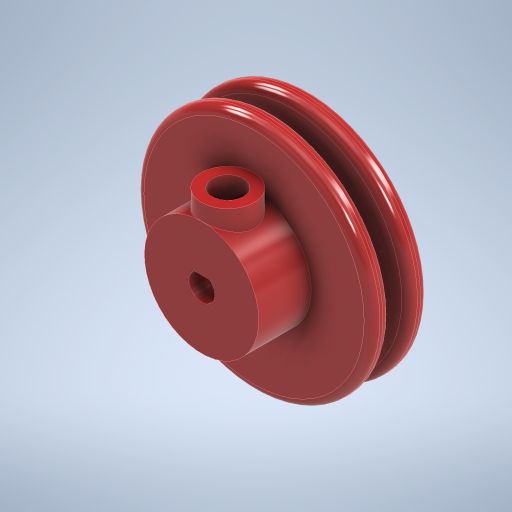
# Autodesk Inventor part: Motor Spool For Door Opener
Saved by Autodesk Inventor 2024 (Build 280153000, 153)
## iProperties
Created: 2024-01-28
Part Number: Motor Spool For Door Opener
Material: ABS Plastic
Document SubType Name: Modeling
Designer: himmelb
Density: 1.06 g/cm^3
Appearance: Red
Author: himmelb
Autodesk Inventor part; units mm, degrees
ref_plane "YZ Plane" through (0, 0, 0) normal (1, 0, 0) x (0, 1, 0)
ref_plane "XZ Plane" through (0, 0, 0) normal (0, 1, 0) x (-1, 0, 0)
sketch "Sketch1" plane through (0, 0, 0) normal (0, 0, 1) x (1, 0, 0)
  circle A0 centre (0, 0) radius 22.5
  dimension "d0" = 45
  constraints: 1 centre point, 1 coincident
  measures "d0" diameter of A0
extrude "Extrusion1" add sketch "Sketch1" against normal blind 3.5833
sketch "Sketch2" plane through (0, 0, -3.5833) normal (0, 0, -1) x (-1, 0, 0)
  circle A0 centre (0, 0) radius 10
  dimension "d14" = 20
  constraints: 1 centre point
  measures "d14" diameter of A0
extrude "Extrusion2" add sketch "Sketch2" along normal blind 3.5833
sketch "Sketch3" plane through (0, 0, -7.1666) normal (0, 0, -1) x (-1, 0, 0)
  circle A0 centre (0, 0) radius 22.5
  dimension "d19" = 45
  constraints: 1 centre point, 1 coincident
  measures "d19" diameter of A0
extrude "Extrusion3" add sketch "Sketch3" along normal blind 3.5833
fillet "Fillet2" radius 1.5 6 edges at (-22.5, 0, 0) (22.5, 0, -7.1666) (22.5, 0, -10.7499) (-22.5, 0, -3.5833) (10, 0, -7.1666) (10, 0, -3.5833)
sketch "Sketch4" plane through (0, 0, 0) normal (0, 0, 1) x (1, 0, 0)
  arc A0 (-1.5033, 2.01) -> (1.5033, 2.01) centre (0, 0) ccw
  line L0 (-1.5033, 2.01) -> (1.5033, 2.01)
  dimension "d15" = 5.02
  constraints: 2 end point, 2 point on circle, 1 centre point, 1 coincident, 1 horizontal
  measures "d15" diameter of A0
extrude "Extrusion4" cut sketch "Sketch4" against normal through all
sketch "Sketch5" plane through (0, 0, 0) normal (0, 0, 1) x (1, 0, 0)
  arc A0 (-1.5033, 2.01) -> (1.5033, 2.01) centre (0, 0) ccw projected
  circle A1 centre (0, 0) radius 10.91
  line L0 (-1.5033, 2.01) -> (1.5033, 2.01) projected
  point P0 (0, 10.91)
  point P1 (0, 2.01)
  dimension "d21" = 21.82
  dimension "d20" = 8.9
  constraints: 1 coincident, 1 midpoint, 1 vertical alignment, 2 other
  measures "d20" distance of point (0, 2.01) point (0, 10.91)
extrude "Extrusion5" add sketch "Sketch5" along normal blind 10
ref_plane "Work Plane1" through (-1.5033, 10.91, -10.7499) normal (0, -1, 0) x (1, 0, 0)
sketch "Sketch10" plane through (-1.5033, 10.91, -10.7499) normal (0, -1, 0) x (1, 0, 0)
  circle A0 centre (1.5033, 15.7499) radius 5
  line L0 (12.4133, 20.7499) -> (-9.4067, 20.7499) projected
  point P0 (1.5033, 10.7499)
  dimension "d40" = 10
  dimension "d51" = 5
  constraints: 1 centre point
  measures "d40" diameter of A0
  measures "d51" distance from line of L0 A0.centre
extrude "Extrusion9" add sketch "Sketch10" along normal mid plane 6.2
sketch "Sketch11" plane through (-1.5033, 14.01, -10.7499) normal (0, 1, 0) x (1, 0, 0)
  circle A0 centre (1.5033, -15.7499) radius 3
  circle A1 centre (1.5033, -15.7499) radius 5 projected
  point P0 (1.5033, -10.7499)
  point P1 (1.2173, -10.7499)
  point P2 (1.7894, -10.7499)
  point P3 (1.5033, -20.7499)
  dimension "d43" = 6
  dimension "d44" = 5
  constraints: 1 centre point, 2 other
  measures "d43" diameter of A0
  measures "d44" distance of point (1.503, -20.75) A0.centre
extrude "Extrusion10" cut sketch "Sketch11" against normal blind 6.8 contours A0
sketch "Sketch12" plane through (0, 7.21, 5) normal (0, 1, 0) x (1, 0, 0)
  circle A0 centre (0, 0) radius 1.335
  circle A1 centre (0, 0) radius 5 projected
  point P0 (0, 5)
  point P1 (-0.2861, 3.9898)
  point P2 (0.2861, 3.9898)
  point P3 (0, -5)
  dimension "d47" = 2.67
  dimension "d48" = 5
  constraints: 1 centre point, 2 other
  measures "d47" diameter of A0
  measures "d48" distance of point (0, -5) A0.centre
extrude "Extrusion11" cut sketch "Sketch12" against normal up to surface (5.2 mm away) contours A0
body "Solid1"
